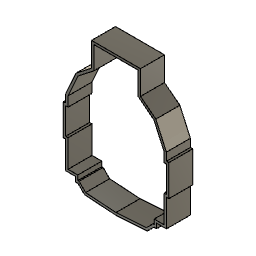
train_clearance_gauge (Autodesk Fusion 360 design; units mm, degrees)
Autodesk Fusion 360 part; units mm, degrees
note: some values were not read from the file. Set by a fixed rule: which face or edge a step refers to.
sketch "Sketch1" plane through (0, 0, 0) normal (0, 1, 0) x (1, 0, 0)
  line L0 (0, 0) -> (131, -9)
  line L1 (131, -9) -> (158, -36)
  line L2 (158, -36) -> (169, -36)
  line L3 (169, -36) -> (169, -56)
  line L4 (169, -56) -> (210, -56)
  line L5 (210, -56) -> (210, -170)
  line L6 (210, -170) -> (220, -170)
  line L7 (220, -170) -> (220, -300)
  line L8 (220, -300) -> (210, -300)
  line L9 (210, -300) -> (210, -333)
  line L10 (210, -333) -> (166, -430)
  line L11 (166, -430) -> (102, -480)
  line L12 (102, -480) -> (102, -580)
  line L13 (102, -580) -> (0, -580)
  line L14 (210, -333) -> (166, -430)
  line L15 (210, -56) -> (210, -170)
  line L16 (102, -480) -> (102, -580)
  line L17 (210, -300) -> (210, -333)
  line L18 (220, -300) -> (210, -300)
  line L19 (131, -9) -> (158, -36)
  line L20 (0, 0) -> (131, -9)
  line L21 (220, -170) -> (220, -300)
  line L22 (102, -580) -> (0, -580)
  line L23 (169, -36) -> (169, -56)
  line L24 (158, -36) -> (169, -36)
  line L25 (166, -430) -> (102, -480)
  line L26 (210, -170) -> (220, -170)
  line L27 (169, -56) -> (210, -56)
  line L28 (-220, -170) -> (-220, -300)
  line L29 (-210, -56) -> (-210, -170)
  line L30 (-210, -56) -> (-210, -170)
  line L31 (-102, -580) -> (0, -580)
  line L32 (-102, -480) -> (-102, -580)
  line L33 (-210, -170) -> (-220, -170)
  line L34 (-210, -333) -> (-166, -430)
  line L35 (-210, -300) -> (-210, -333)
  line L36 (-220, -300) -> (-210, -300)
  line L37 (-169, -56) -> (-210, -56)
  line L38 (-158, -36) -> (-169, -36)
  line L39 (-166, -430) -> (-102, -480)
  line L40 (-210, -333) -> (-166, -430)
  line L41 (-102, -580) -> (0, -580)
  line L42 (-220, -300) -> (-210, -300)
  line L43 (-102, -480) -> (-102, -580)
  line L44 (-220, -170) -> (-220, -300)
  line L45 (-131, -9) -> (-158, -36)
  line L46 (-169, -36) -> (-169, -56)
  line L47 (-210, -300) -> (-210, -333)
  line L48 (-131, -9) -> (-158, -36)
  line L49 (-166, -430) -> (-102, -480)
  line L50 (-169, -36) -> (-169, -56)
  line L51 (-169, -56) -> (-210, -56)
  line L52 (-210, -170) -> (-220, -170)
  line L53 (0, 0) -> (-131, -9)
  line L54 (-158, -36) -> (-169, -36)
  line L55 (0, 0) -> (-131, -9)
  dimension "d5" = 11
  dimension "d6" = 20
  dimension "d7" = 41
  dimension "d8" = 114
  dimension "d9" = 130
  dimension "d10" = 10
  dimension "d11" = 33
  dimension "d16" = 100
  dimension "d17" = 11
  dimension "d18" = 20
  dimension "d19" = 41
  dimension "d20" = 114
  dimension "d21" = 130
  dimension "d22" = 10
  dimension "d23" = 33
  dimension "d24" = 100
  constraint coincident L0.start L20.start
  constraint horizontal L2
  constraint perpendicular L2 L3
  constraint perpendicular L3 L4
  constraint perpendicular L4 L5
  constraint perpendicular L5 L6
  constraint perpendicular L6 L7
  constraint perpendicular L7 L8
  constraint perpendicular L8 L9
  constraint vertical L12
  constraint perpendicular L12 L13
  constraint horizontal L24
  constraint perpendicular L23 L24
  constraint perpendicular L23 L27
  constraint perpendicular L15 L27
  constraint perpendicular L15 L26
  constraint perpendicular L21 L26
  constraint perpendicular L18 L21
  constraint perpendicular L17 L18
  constraint vertical L16
  constraint perpendicular L16 L22
  measures "d5" distance of L1.end L2.end
  measures "d6" distance of L2.end L3.end
  measures "d7" distance of L3.end L4.end
  measures "d8" distance of L4.end L5.end
  measures "d9" distance of L6.end L7.end
  measures "d10" distance of L7.end L8.end
  measures "d11" distance of L8.end L9.end
  measures "d16" distance of L11.end L12.end
  measures "d17" distance of L2.end L1.end
  measures "d18" distance of L3.end L2.end
  measures "d19" distance of L4.end L3.end
  measures "d20" distance of L5.end L4.end
  measures "d21" distance of L7.end L6.end
  measures "d22" distance of L8.end L7.end
  measures "d23" distance of L8.end L9.end
  measures "d24" distance of L11.end L12.end
extrude "Extrude1" add sketch "Sketch1" along normal blind 100
shell "Shell1" thickness 10 removed faces 1 at (-34, 100, 360)
delete_face "DeleteFace1" 1 faces at (30.6667, 10, 351.7075)
